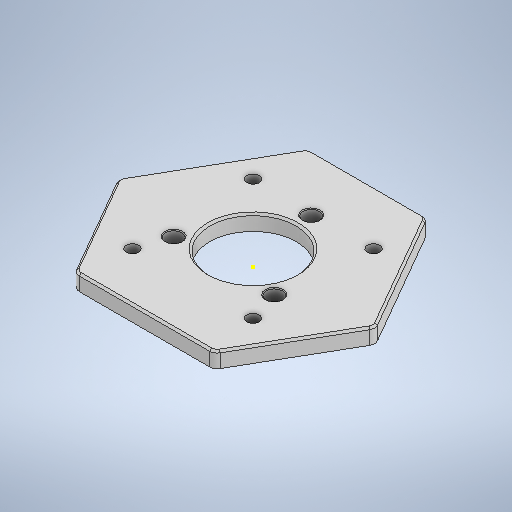
# Autodesk Inventor part: 4_DOF
Saved by Autodesk Inventor 2025 (Build 290162000, 162)
## iProperties
Created: 2026-06-13
Part Number: 4_DOF
Material: Generic
Document SubType Name: Sheet Metal
Designer: MSI
Density: 1 g/cm^3
Sheet Metal Rule: Default_mm
Appearance: Default
Author: MSI
Autodesk Inventor part; units mm, degrees
ref_plane "YZ Plane" through (0, 0, 0) normal (1, 0, 0) x (0, 1, 0)
ref_plane "XZ Plane" through (0, 0, 0) normal (0, 1, 0) x (-1, 0, 0)
ref_plane "XY Plane" through (0, 0, 0) normal (0, 0, 1) x (1, 0, 0)
sketch "Sketch1" plane through (0, 0, 0) normal (0, 1, 0) x (-1, 0, 0)
  circle A0 centre (0, -15) radius 2.1
  circle A1 centre (12.9904, 7.5) radius 2.1
  circle A2 centre (-12.9904, 7.5) radius 2.1
  line L0 (20.4449, 23.6603) -> (30.7128, 5.8756)
  line L1 (-20.4449, 23.6603) -> (-30.7128, 5.8756)
  line L2 (-10.2679, -29.5359) -> (10.2679, -29.5359)
  circle A3 centre (15.55, -15.55) radius 1.6
  circle A4 centre (15.55, 15.55) radius 1.6
  circle A5 centre (-15.55, 15.55) radius 1.6
  circle A6 centre (-15.55, -15.55) radius 1.6
  line L3 (30.7128, 5.8756) -> (33.2128, 1.5455)
  line L4 (-20.4449, 23.6603) -> (-17.9449, 27.9904)
  line L5 (-10.2679, -29.5359) -> (-15.2679, -29.5359)
  line L6 (10.2679, -29.5359) -> (15.2679, -29.5359)
  line L7 (20.4449, 23.6603) -> (17.9449, 27.9904)
  line L8 (-30.7128, 5.8756) -> (-33.2128, 1.5455)
  line L9 (17.9449, 27.9904) -> (-17.9449, 27.9904)
  line L10 (15.2679, -29.5359) -> (33.2128, 1.5455)
  line L11 (17.9449, 27.9904) -> (-17.9449, 27.9904)
  line L12 (-33.2128, 1.5455) -> (-15.2679, -29.5359)
  circle A7 centre (0, 0) radius 11.15
  dimension "d29" = 360
  dimension "d77" = 360
  dimension "d82" = 360
  dimension "d86" = 360
  dimension "d90" = 360
  constraints: 26 end point, 8 centre point, 3 coincident, 2 horizontal, 47 other
sketch "Sketch4" plane through (0, 0, 0) normal (0, 1, 0) x (-1, 0, 0)
  point P0 (0, 0)
extrude "Extrusion5" add sketch "Sketch1" along normal blind 4
chamfer "Chamfer6" distance 0.5 angle 45 1 edges at (11.15, 4, 0)
chamfer "Chamfer7" distance 0.2 angle 45 3 edges at (-10.8904, 4, 7.5) (2.1, 4, -15) (15.0904, 4, 7.5)
fillet "Fillet1" radius 2 6 edges at (17.9449, 2, 27.9904) (33.2128, 2, 1.5455) (15.2679, 2, -29.5359) (-15.2679, 2, -29.5359) (-33.2128, 2, 1.5455) (-17.9449, 2, 27.9904)
chamfer "Chamfer8" distance 0.5 angle 45 18 edges at (-24.2404, 4, -13.9952) (-32.9034, 4, 1.5455) (-19.4835, 4, 25.3253) (-25.5788, 4, 14.7679) (-31.6741, 4, 4.2106) (-17.7902, 4, 27.7224) (0, 4, 27.9904) (17.7902, 4, 27.7224) (19.4835, 4, 25.3253) (25.5788, 4, 14.7679) (31.6741, 4, 4.2106) (32.9034, 4, 1.5455) (24.2404, 4, -13.9952) (15.1132, 4, -29.2679) (-12.1906, 4, -29.5359) (0, 4, -29.5359) (12.1906, 4, -29.5359) (-15.1132, 4, -29.2679)
equation "\"BendRadius\" = Thickness"
equation "\"BendReliefWidth\" = Thickness"
equation "\"BendReliefDepth\" = 0.5 * Thickness"
equation "\"CornerReliefSize\" = 4 * Thickness"
equation "\"MinimumRemnant\" = 2 * Thickness"
equation "\"TransitionRadius\" = BendRadius"
equation "\"JacobiRadiusSize\" = BendRadius"
equation "\"GapSize\" = Thickness"
equation "\"Thickness\" = 0.5"
body "Solid2"
